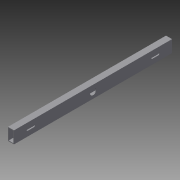
# Autodesk Inventor part: frame_long
Saved by Autodesk Inventor 2015 SP1 (Build 190203100, 203)
## iProperties
Created: 2014-12-28
Part Number: frame_long
Material: Generic
Document SubType Name: Modeling
Designer: Jarod
Density: 1 g/cm^3
Appearance: Default
Author: Jarod
Autodesk Inventor part; units mm, degrees
ref_plane "YZ Plane" through (0, 0, 0) normal (1, 0, 0) x (0, 1, 0)
ref_plane "XZ Plane" through (0, 0, 0) normal (0, 1, 0) x (-1, 0, 0)
ref_plane "XY Plane" through (0, 0, 0) normal (0, 0, 1) x (1, 0, 0)
sketch "Sketch1" plane through (0, 0, 0) normal (0, 0, 1) x (1, 0, 0)
  line L0 (0, 0) -> (25.4, 0)
  line L1 (25.4, 0) -> (25.4, 50.8)
  line L2 (25.4, 50.8) -> (0, 50.8)
  line L3 (0, 50.8) -> (0, 0)
  line L4 (3.175, 3.175) -> (22.225, 3.175)
  line L5 (22.225, 3.175) -> (22.225, 47.625)
  line L6 (22.225, 47.625) -> (3.175, 47.625)
  line L7 (3.175, 47.625) -> (3.175, 3.175)
  dimension "d0" = 25.4
  dimension "d1" = 50.8
  dimension "d2" = 19.05
  dimension "d3" = 44.45
  dimension "d4" = 3.175
  dimension "d5" = 3.175
  constraints: 16 end point, 4 parallel, 2 horizontal, 2 perpendicular
  measures "d0" distance of L2.end L1.end
  measures "d1" distance of L1.end L0.end
  measures "d2" distance of L6.end L5.end
  measures "d3" distance of L5.end L4.end
  measures "d4" distance between parallel lines of L0 L4
  measures "d5" distance between parallel lines of L3 L7
extrude "Extrusion1" add sketch "Sketch1" along normal blind 660.4
sketch "Sketch2" plane through (25.4, 0, 0) normal (1, 0, 0) x (0, 0, -1)
  line L0 (0, 0) -> (0, 50.8) projected
  line L1 (0, 50.8) -> (-660.4, 50.8) projected
  line L2 (-660.4, 0) -> (-660.4, 50.8) projected
  line L3 (0, 0) -> (-660.4, 0) projected
  circle A0 centre (-330.2, 25.4) radius 12.7
  line L4 (-603.25, 25.4) -> (-603.25, 20.6375) construction
  line L5 (-603.25, 20.6375) -> (-603.25, 30.1625) construction
  line L6 (-577.85, 25.4) -> (-577.85, 20.6375) construction
  line L7 (-577.85, 20.6375) -> (-577.85, 30.1625) construction
  line L8 (-82.55, 25.4) -> (-82.55, 20.6375) construction
  line L9 (-82.55, 25.4) -> (-77.7875, 25.4) construction
  line L10 (-82.55, 20.6375) -> (-82.55, 30.1625) construction
  line L11 (-57.15, 25.4) -> (-57.15, 20.6375) construction
  line L12 (-57.15, 25.4) -> (-52.3875, 25.4) construction
  line L13 (-57.15, 20.6375) -> (-57.15, 30.1625) construction
  arc A1 (-603.25, 30.1625) -> (-603.25, 20.6375) centre (-603.047, 25.4) ccw
  arc A2 (-577.85, 20.6375) -> (-577.85, 30.1625) centre (-577.2085, 25.4) ccw
  arc A3 (-82.55, 30.1625) -> (-82.55, 20.6375) centre (-81.7597, 25.4) ccw
  arc A4 (-57.15, 20.6375) -> (-57.15, 30.1625) centre (-57.2051, 25.4) ccw
  line L14 (-82.55, 30.1625) -> (-57.15, 30.1625)
  line L15 (-57.15, 20.6375) -> (-82.55, 20.6375)
  line L16 (-603.25, 30.1625) -> (-577.85, 30.1625)
  line L17 (-577.85, 20.6375) -> (-603.25, 20.6375)
  dimension "d8" = 25.4
  dimension "d9" = 330.2
  dimension "d10" = 25.4
  dimension "d11" = 25.4
  dimension "d12" = 25.4
  dimension "d13" = 25.4
  dimension "d14" = 25.4
  dimension "d15" = 57.15
  dimension "d16" = 57.15
  dimension "d17" = 82.55
  dimension "d18" = 82.55
  dimension "d19" = 4.7625
  dimension "d20" = 9.525
  dimension "d21" = 4.7625
  dimension "d22" = 9.525
  dimension "d23" = 4.7625
  dimension "d24" = 90
  dimension "d25" = 9.525
  dimension "d26" = 4.7625
  dimension "d27" = 90
  dimension "d28" = 9.525
  dimension "d29" = 4.7668
  dimension "d30" = 4.8055
  dimension "d31" = 4.8276
  dimension "d32" = 4.7628
  constraints: 28 end point, 8 point on circle, 5 centre point, 4 point on line, 4 vertical, 2 horizontal, 2 perpendicular, 1 coincident
  measures "d8" distance from line of L3 point (-330.2, 25.4)
  measures "d9" distance from line of L2 point (-330.2, 25.4)
  measures "d10" diameter of A0
  measures "d11" distance from line of L3 L4.start
  measures "d12" distance from line of L3 L6.start
  measures "d13" distance from line of L3 L8.start
  measures "d14" distance from line of L3 L11.start
  measures "d15" distance from line of L0 L11.start
  measures "d16" distance from line of L4.start L2
  measures "d17" distance from line of L6.start L2
  measures "d18" distance from line of L8.start L0
  measures "d19" distance of L4.start L4.end
  measures "d20" distance of L4.end L5.end
  measures "d21" distance of L6.start L6.end
  measures "d22" distance of L6.end L7.end
  measures "d23" distance of L8.start L8.end
  measures "d24" angle of L8 L9
  measures "d25" distance of L8.end L10.end
  measures "d26" distance of L11.start L11.end
  measures "d27" angle of L11 L12
  measures "d28" distance of L11.end L13.end
  measures "d29" radius of A1
  measures "d30" radius of A2
  measures "d31" radius of A3
  measures "d32" radius of A4
extrude "Extrusion2" cut sketch "Sketch2" against normal blind 762 contours A0 | L16 A2 L17 A1 | L14 A4 L15 A3
body "Solid1"
